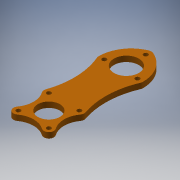
# Autodesk Inventor part: Part69
Saved by Autodesk Inventor 2017 SP1 (Build 210196100, 196)
## iProperties
Created: 2018-01-30
Part Number: Part69
Material: Aluminum 6061
Document SubType Name: Modeling
Designer: Ben
Density: 2.7 g/cm^3
Appearance: Orange
Author: Ben
Autodesk Inventor part; units mm, degrees
ref_plane "YZ Plane" through (0, 0, 0) normal (1, 0, 0) x (0, 1, 0)
ref_plane "XZ Plane" through (0, 0, 0) normal (0, 1, 0) x (-1, 0, 0)
ref_plane "XY Plane" through (0, 0, 0) normal (0, 0, 1) x (1, 0, 0)
sketch "Sketch1" plane through (0, 0, 0) normal (0, 1, 0) x (-1, 0, 0)
  circle A0 centre (0, 0) radius 14.2875
  line L0 (143.7805, 15.875) -> (-143.7805, 15.875) construction
  line L1 (0, 0) -> (0, 15.875) construction
  circle A1 centre (0, 88.9254) radius 12.7
  line L2 (0, 15.875) -> (0, 88.9254) construction
  line L3 (17.4625, 71.4629) -> (-17.4625, 106.3879) construction
  line L4 (17.4625, 106.3879) -> (-17.4625, 71.4629) construction
  circle A2 centre (17.4625, 71.4629) radius 2.4892
  circle A3 centre (-17.4625, 106.3879) radius 2.4892
  circle A4 centre (-17.4625, 71.4629) radius 2.4892
  circle A5 centre (17.4625, 106.3879) radius 2.4892
  circle A6 centre (0, 0) radius 50.8 construction
  line L5 (143.7805, -34.925) -> (-143.7805, -34.925) construction
  line L6 (0, 0) -> (0, -34.925) construction
  circle A7 centre (19.05, 6.35) radius 2.54
  circle A8 centre (-19.05, 6.35) radius 2.54
  circle A9 centre (0, -22.225) radius 2.54
  line L7 (19.05, 6.35) -> (-19.05, 6.35) construction
  arc A10 (-2.4454, -28.0852) -> (2.4454, -28.0852) centre (0, -22.225) ccw
  arc A11 (-24.9019, 8.8154) -> (-25.4, 6.3466) centre (-19.05, 6.35) ccw
  arc A12 (25.4, 6.3466) -> (24.9019, 8.8154) centre (19.05, 6.35) ccw
  arc A13 (22.0483, 103.0632) -> (14.1378, 110.9737) centre (17.4625, 106.3879) ccw
  arc A14 (-14.1378, 110.9737) -> (-22.0483, 103.0632) centre (-17.4625, 106.3879) ccw
  arc A15 (-22.0483, 74.7876) -> (-22.8205, 69.6258) centre (-17.4625, 71.4629) ccw
  arc A16 (22.8205, 69.6258) -> (22.0483, 74.7876) centre (17.4625, 71.4629) ccw
  arc A17 (-14.1378, 110.9737) -> (14.1378, 110.9737) centre (0, 130.4739) ccw
  arc A18 (22.0483, 103.0632) -> (22.0483, 74.7876) centre (41.5485, 88.9254) ccw
  arc A19 (-22.0483, 74.7876) -> (-22.0483, 103.0632) centre (-41.5485, 88.9254) ccw
  arc A20 (22.8205, 69.6258) -> (24.9019, 8.8154) centre (103.546, 41.948) ccw
  arc A21 (-24.9019, 8.8154) -> (-22.8205, 69.6258) centre (-103.546, 41.948) ccw
  line L8 (19.05, 6.35) -> (17.4625, 71.4629) construction
  line L9 (-17.4625, 71.4629) -> (-19.05, 6.35) construction
  arc A22 (2.4454, -28.0852) -> (25.4, 6.3466) centre (-11.9308, 6.3664) ccw
  arc A23 (-25.4, 6.3466) -> (-2.4454, -28.0852) centre (11.9308, 6.3664) ccw
  line L10 (12.3733, -7.1438) -> (20.6222, -11.9063) construction
  point P0 (0, 6.35)
  dimension "d0" = 28.575
  dimension "d1" = 15.875
  dimension "d2" = 34.925
  dimension "d3" = 4.9784
  dimension "d4" = 88.9254
  dimension "d5" = 101.6
  dimension "d6" = 25.4
  dimension "d7" = 50.8
  dimension "d8" = 5.08
  dimension "d9" = 9.525
  dimension "d10" = 38.1
  dimension "d12" = 6.35
  dimension "d13" = 3.175
  dimension "d14" = 4.7625
  dimension "d18" = 28.575
  dimension "d19" = 9.525
  dimension "d20" = 60
  constraints: 29 point on circle, 23 centre point, 22 end point, 15 tangent, 14 equal radius, 13 coincident, 5 midpoint, 3 horizontal, 3 point on line, 2 equal length, 2 perpendicular, 2 vertical, 4 other
  measures "d1" distance of L1.start L1.end
  measures "d2" distance of L4.start L3.start
  measures "d3" diameter of A2
  measures "d4" distance of L2.end point (0, 0)
  measures "d5" diameter of A6
  measures "d6" diameter of A1
  measures "d7" distance between parallel lines of L0 L5
  measures "d8" diameter of A7
  measures "d9" distance between parallel lines of L0 L7
  measures "d10" distance of L7.start L7.end
  measures "d12" radius of A10
  measures "d13" radial gap between concentric circles of A5 A13
  measures "d18" distance from line of L7 A9.centre
  measures "d19" distance of L10.start L10.end
  measures "d20" angle of L6 L10
extrude "Extrusion1" add sketch "Sketch1" along normal blind 6.35
body "Solid1"
